Autodesk Inventor part; units mm, degrees
(part 3 of 3)
sketch "Sketch1 outline for Extrusion2" plane through (0, 0, 0) normal (0, 0, 1) x (1, 0, 0)
  arc A0 (21.457911, 5.391973) -> (21.768736, 3.954452) centre (0.000012, -0.000078) cw
  spline S0 degree 3 poles (18.997609, 5.539001) (19.076402, 5.554495) (19.252325, 5.587248) (19.530013, 5.604888) (19.826012, 5.602764) (20.12188, 5.590993) (20.417028, 5.567223) (20.711048, 5.532217) (21.003535, 5.486112) (21.252244, 5.437621) (21.40332, 5.404433) (21.457911, 5.391973) knots 0 0 0 0 0.0970257 0.21631999 0.33564552 0.45497381 0.57430193 0.69363012 0.81295881 0.93228849 1 1 1 1
  spline S1 degree 3 poles (21.768736, 3.954452) (21.724169, 3.920552) (21.600299, 3.827915) (21.39384, 3.681006) (21.146528, 3.518184) (20.893235, 3.364836) (20.634271, 3.221255) (20.369696, 3.088303) (20.101015, 2.964082) (19.840845, 2.865426) (19.667105, 2.822573) (19.588951, 2.804131) knots 0 0 0 0 0.06771151 0.18704119 0.30636988 0.42569807 0.54502619 0.66435448 0.78368001 0.9029743 1 1 1 1
  arc A1 (18.32817, 5.932845) -> (18.997609, 5.539001) centre (18.884737, 6.113009) ccw
  arc A2 (19.588951, 2.804131) -> (19.14202, 2.168903) centre (19.723301, 2.234768) ccw
  arc A3 (18.179447, 6.374019) -> (18.32817, 5.932845) centre (0.000012, -0.000078) cw
  arc A4 (19.14202, 2.168903) -> (19.188845, 1.705696) centre (0.000012, -0.000078) cw
  arc A5 (18.47382, 7.092773) -> (18.179447, 6.374019) centre (18.731497, 6.56758) ccw
  arc A6 (19.188845, 1.705696) -> (19.753861, 1.172762) centre (19.771547, 1.757495) ccw
  spline S2 degree 3 poles (20.342983, 8.6993) (20.307077, 8.656333) (20.206926, 8.538455) (20.038334, 8.349288) (19.833454, 8.135517) (19.620634, 7.92965) (19.400113, 7.732044) (19.171756, 7.543552) (18.937454, 7.362659) (18.70576, 7.208582) (18.545911, 7.128143) (18.47382, 7.092773) knots 0 0 0 0 0.06771151 0.18704119 0.30636988 0.42569807 0.54502619 0.66435448 0.78368001 0.9029743 1 1 1 1
  spline S3 degree 3 poles (19.753861, 1.172762) (19.834125, 1.170334) (20.012926, 1.163119) (20.287577, 1.118526) (20.575682, 1.050589) (20.861513, 0.973276) (21.143972, 0.884426) (21.422831, 0.784871) (21.697725, 0.674838) (21.929408, 0.57222) (22.069312, 0.506247) (22.11976, 0.481952) knots 0 0 0 0 0.0970257 0.21631999 0.33564552 0.45497381 0.57430193 0.69363012 0.81295881 0.93228849 1 1 1 1
  arc A7 (19.720072, 10.031615) -> (20.342983, 8.6993) centre (0.000012, -0.000078) cw
  arc A8 (22.11976, 0.481952) -> (22.102914, -0.988693) centre (0.000012, -0.000078) cw
  spline S4 degree 3 poles (17.288739, 9.627488) (17.362108, 9.660126) (17.526333, 9.731205) (17.793133, 9.810194) (18.082183, 9.873989) (18.373252, 9.92835) (18.66629, 9.970853) (18.960728, 10.00215) (19.256141, 10.022285) (19.509404, 10.030353) (19.664078, 10.031615) (19.720072, 10.031615) knots 0 0 0 0 0.0970257 0.21631999 0.33564552 0.45497381 0.57430193 0.69363012 0.81295881 0.93228849 1 1 1 1
  spline S5 degree 3 poles (22.102914, -0.988693) (22.051921, -1.011826) (21.910543, -1.074577) (21.67657, -1.171861) (21.399228, -1.275568) (21.118162, -1.368709) (20.833741, -1.451065) (20.546215, -1.52181) (20.256629, -1.58313) (19.981028, -1.621419) (19.802109, -1.624537) (19.72181, -1.625125) knots 0 0 0 0 0.06771151 0.18704119 0.30636988 0.42569807 0.54502619 0.66435448 0.78368001 0.9029743 1 1 1 1
  arc A9 (16.548445, 9.862494) -> (17.288739, 9.627488) centre (17.050967, 10.161988) ccw
  arc A10 (19.72181, -1.625125) -> (19.144734, -2.144976) centre (19.726097, -2.210109) ccw
  arc A11 (16.30528, 10.259512) -> (16.548445, 9.862494) centre (0.000012, -0.000078) cw
  arc A12 (19.144734, -2.144976) -> (19.087311, -2.606988) centre (0.000012, -0.000078) cw
  arc A13 (16.432335, 11.025749) -> (16.30528, 10.259512) centre (16.800418, 10.571063) ccw
  arc A14 (19.087311, -2.606988) -> (19.519572, -3.252288) centre (19.66693, -2.686152) ccw
  spline S6 degree 3 poles (17.897148, 13.007925) (17.871704, 12.958046) (17.800294, 12.820837) (17.678023, 12.598898) (17.525848, 12.344896) (17.364174, 12.096835) (17.193153, 11.855112) (17.012465, 11.620532) (16.824289, 11.392037) (16.63269, 11.190266) (16.494749, 11.076275) (16.432335, 11.025749) knots 0 0 0 0 0.06771151 0.18704119 0.30636988 0.42569807 0.54502619 0.66435448 0.78368001 0.9029743 1 1 1 1
  spline S7 degree 3 poles (19.519572, -3.252288) (19.597284, -3.272516) (19.769996, -3.319337) (20.027838, -3.423928) (20.293603, -3.554271) (20.555063, -3.693249) (20.81067, -3.842724) (21.060383, -4.001835) (21.303901, -4.170279) (21.50694, -4.321878) (21.628656, -4.417329) (21.672434, -4.452241) knots 0 0 0 0 0.0970257 0.21631999 0.33564552 0.45497381 0.57430193 0.69363012 0.81295881 0.93228849 1 1 1 1
  arc A15 (16.993387, 14.168226) -> (17.897148, 13.007925) centre (0.000012, -0.000078) cw
  arc A16 (21.672434, -4.452241) -> (21.32876, -5.882265) centre (0.000012, -0.000078) cw
  spline S8 degree 3 poles (14.712939, 13.233209) (14.777206, 13.281355) (14.921497, 13.387194) (15.164031, 13.523572) (15.431639, 13.650087) (15.703314, 13.767854) (15.979547, 13.874499) (16.259638, 13.970529) (16.543164, 14.055895) (16.788282, 14.120117) (16.938797, 14.155766) (16.993387, 14.168226) knots 0 0 0 0 0.0970257 0.21631999 0.33564552 0.45497381 0.57430193 0.69363012 0.81295881 0.93228849 1 1 1 1
  spline S9 degree 3 poles (21.32876, -5.882265) (21.273899, -5.893471) (21.122102, -5.923189) (20.872347, -5.96597) (20.578881, -6.005363) (20.284137, -6.033625) (19.988521, -6.050627) (19.692461, -6.055617) (19.396491, -6.05096) (19.11928, -6.026963) (18.944153, -5.990189) (18.865736, -5.972895) knots 0 0 0 0 0.06771151 0.18704119 0.30636988 0.42569807 0.54502619 0.66435448 0.78368001 0.9029743 1 1 1 1
  arc A17 (13.938913, 13.297591) -> (14.712939, 13.233209) centre (14.362192, 13.701398) ccw
  arc A18 (18.865736, -5.972895) -> (18.187451, -6.3513) centre (18.739744, -6.544166) ccw
  arc A19 (13.6135, 13.630547) -> (13.938913, 13.297591) centre (0.000012, -0.000078) cw
  arc A20 (18.187451, -6.3513) -> (18.02866, -6.788951) centre (0.000012, -0.000078) cw
  arc A21 (13.566865, 14.405845) -> (13.6135, 13.630547) centre (14.026897, 14.044464) ccw
  arc A22 (18.02866, -6.788951) -> (18.306491, -7.514259) centre (18.576131, -6.995107) ccw
  spline S10 degree 3 poles (14.553877, 16.664275) (14.54017, 16.609984) (14.501082, 16.460326) (14.431262, 16.216743) (14.339423, 15.935247) (14.237002, 15.657429) (14.124057, 15.383712) (14.000098, 15.114806) (13.867486, 14.850166) (13.725588, 14.61082) (13.616471, 14.468992) (13.566865, 14.405845) knots 0 0 0 0 0.06771151 0.18704119 0.30636988 0.42569807 0.54502619 0.66435448 0.78368001 0.9029743 1 1 1 1
  spline S11 degree 3 poles (18.306491, -7.514259) (18.377753, -7.551272) (18.535717, -7.635352) (18.763821, -7.794695) (18.993918, -7.980909) (19.217897, -8.174582) (19.433834, -8.377188) (19.641881, -8.587876) (19.841811, -8.806284) (20.006025, -8.999264) (20.10345, -9.119405) (20.138362, -9.163183) knots 0 0 0 0 0.0970257 0.21631999 0.33564552 0.45497381 0.57430193 0.69363012 0.81295881 0.93228849 1 1 1 1
  arc A23 (13.414584, 17.594379) -> (14.553877, 16.664275) centre (0.000012, -0.000078) cw
  arc A24 (20.138362, -9.163183) -> (19.485094, -10.480879) centre (0.000012, -0.000078) cw
  spline S12 degree 3 poles (11.399372, 16.175357) (11.451315, 16.236597) (11.568436, 16.37189) (11.774542, 16.558818) (12.007288, 16.741709) (12.245947, 16.916976) (12.491523, 17.082415) (12.743223, 17.238364) (13.000644, 17.38468) (13.225326, 17.501836) (13.364135, 17.570084) (13.414584, 17.594379) knots 0 0 0 0 0.0970257 0.21631999 0.33564552 0.45497381 0.57430193 0.69363012 0.81295881 0.93228849 1 1 1 1
  spline S13 degree 3 poles (19.485094, -10.480879) (19.429115, -10.479597) (19.27451, -10.474791) (19.021498, -10.460924) (18.726624, -10.434027) (18.432981, -10.395993) (18.140994, -10.346788) (17.851246, -10.285774) (17.563733, -10.215375) (17.298812, -10.130294) (17.136259, -10.055473) (17.063657, -10.021162) knots 0 0 0 0 0.06771151 0.18704119 0.30636988 0.42569807 0.54502619 0.66435448 0.78368001 0.9029743 1 1 1 1
  arc A25 (10.630426, 16.065888) -> (11.399372, 16.175357) centre (10.953237, 16.553759) ccw
  arc A26 (17.063657, -10.021162) -> (16.318174, -10.239147) centre (16.813703, -10.550075) ccw
  arc A27 (10.239082, 16.318084) -> (10.630426, 16.065888) centre (0.000012, -0.000078) cw
  arc A28 (16.318174, -10.239147) -> (16.065978, -10.630492) centre (0.000012, -0.000078) cw
  arc A29 (10.021097, 17.063567) -> (10.239082, 16.318084) centre (10.550009, 16.813614) ccw
  arc A30 (16.065978, -10.630492) -> (16.175447, -11.399438) centre (16.553849, -10.953303) ccw
  spline S14 degree 3 poles (10.480814, 19.485004) (10.479531, 19.429025) (10.474726, 19.274421) (10.460858, 19.021409) (10.433961, 18.726535) (10.395928, 18.432891) (10.346723, 18.140904) (10.285709, 17.851156) (10.215309, 17.563643) (10.130228, 17.298722) (10.055407, 17.136169) (10.021097, 17.063567) knots 0 0 0 0 0.06771151 0.18704119 0.30636988 0.42569807 0.54502619 0.66435448 0.78368001 0.9029743 1 1 1 1
  spline S15 degree 3 poles (16.175447, -11.399438) (16.236686, -11.45138) (16.37198, -11.568502) (16.558907, -11.774608) (16.741799, -12.007354) (16.917066, -12.246012) (17.082505, -12.491589) (17.238454, -12.743289) (17.38477, -13.00071) (17.501926, -13.225392) (17.570173, -13.3642) (17.594468, -13.414649) knots 0 0 0 0 0.0970257 0.21631999 0.33564552 0.45497381 0.57430193 0.69363012 0.81295881 0.93228849 1 1 1 1
  arc A31 (9.163118, 20.138272) -> (10.480814, 19.485004) centre (0.000012, -0.000078) cw
  arc A32 (17.594468, -13.414649) -> (16.664365, -14.553942) centre (0.000012, -0.000078) cw
  spline S16 degree 3 poles (7.514194, 18.306401) (7.551207, 18.377664) (7.635286, 18.535627) (7.794629, 18.763731) (7.980843, 18.993828) (8.174517, 19.217807) (8.377123, 19.433744) (8.58781, 19.641792) (8.806219, 19.841721) (8.999198, 20.005936) (9.11934, 20.10336) (9.163118, 20.138272) knots 0 0 0 0 0.0970257 0.21631999 0.33564552 0.45497381 0.57430193 0.69363012 0.81295881 0.93228849 1 1 1 1
  spline S17 degree 3 poles (16.664365, -14.553942) (16.610074, -14.540235) (16.460416, -14.501148) (16.216833, -14.431328) (15.935337, -14.339489) (15.657519, -14.237067) (15.383802, -14.124123) (15.114896, -14.000164) (14.850256, -13.867551) (14.61091, -13.725654) (14.469082, -13.616536) (14.405934, -13.566931) knots 0 0 0 0 0.06771151 0.18704119 0.30636988 0.42569807 0.54502619 0.66435448 0.78368001 0.9029743 1 1 1 1
  arc A33 (6.788886, 18.02857) -> (7.514194, 18.306401) centre (6.995042, 18.576042) ccw
  arc A34 (14.405934, -13.566931) -> (13.630636, -13.613565) centre (14.044554, -14.026962) ccw
  arc A35 (6.351234, 18.187361) -> (6.788886, 18.02857) centre (0.000012, -0.000078) cw
  arc A36 (13.630636, -13.613565) -> (13.297681, -13.938979) centre (0.000012, -0.000078) cw
  arc A37 (5.972829, 18.865647) -> (6.351234, 18.187361) centre (6.5441, 18.739654) ccw
  arc A38 (13.297681, -13.938979) -> (13.233298, -14.713005) centre (13.701488, -14.362258) ccw
  spline S18 degree 3 poles (5.882199, 21.32867) (5.893406, 21.273809) (5.923123, 21.122012) (5.965904, 20.872258) (6.005297, 20.578791) (6.033559, 20.284047) (6.050561, 19.988431) (6.055552, 19.692372) (6.050895, 19.396401) (6.026898, 19.119191) (5.990123, 18.944064) (5.972829, 18.865647) knots 0 0 0 0 0.06771151 0.18704119 0.30636988 0.42569807 0.54502619 0.66435448 0.78368001 0.9029743 1 1 1 1
  spline S19 degree 3 poles (13.233298, -14.713005) (13.281444, -14.777272) (13.387284, -14.921563) (13.523662, -15.164097) (13.650177, -15.431705) (13.767944, -15.70338) (13.874588, -15.979613) (13.970619, -16.259704) (14.055985, -16.54323) (14.120207, -16.788348) (14.155856, -16.938863) (14.168315, -16.993453) knots 0 0 0 0 0.0970257 0.21631999 0.33564552 0.45497381 0.57430193 0.69363012 0.81295881 0.93228849 1 1 1 1
  arc A39 (4.452175, 21.672344) -> (5.882199, 21.32867) centre (0.000012, -0.000078) cw
  arc A40 (14.168315, -16.993453) -> (13.008015, -17.897214) centre (0.000012, -0.000078) cw
  spline S20 degree 3 poles (3.252223, 19.519482) (3.27245, 19.597194) (3.319271, 19.769907) (3.423862, 20.027749) (3.554205, 20.293513) (3.693183, 20.554973) (3.842659, 20.81058) (4.001769, 21.060294) (4.170213, 21.303811) (4.321813, 21.50685) (4.417263, 21.628566) (4.452175, 21.672344) knots 0 0 0 0 0.0970257 0.21631999 0.33564552 0.45497381 0.57430193 0.69363012 0.81295881 0.93228849 1 1 1 1
  spline S21 degree 3 poles (13.008015, -17.897214) (12.958136, -17.87177) (12.820927, -17.80036) (12.598988, -17.678088) (12.344986, -17.525914) (12.096924, -17.364239) (11.855202, -17.193219) (11.620622, -17.01253) (11.392126, -16.824355) (11.190356, -16.632755) (11.076365, -16.494814) (11.025839, -16.432401) knots 0 0 0 0 0.06771151 0.18704119 0.30636988 0.42569807 0.54502619 0.66435448 0.78368001 0.9029743 1 1 1 1
  arc A41 (2.606923, 19.087221) -> (3.252223, 19.519482) centre (2.686086, 19.66684) ccw
  arc A42 (11.025839, -16.432401) -> (10.259602, -16.305346) centre (10.571152, -16.800484) ccw
  arc A43 (2.14491, 19.144644) -> (2.606923, 19.087221) centre (0.000012, -0.000078) cw
  arc A44 (10.259602, -16.305346) -> (9.862583, -16.548511) centre (0.000012, -0.000078) cw
  arc A45 (1.625059, 19.72172) -> (2.14491, 19.144644) centre (2.210044, 19.726007) ccw
  arc A46 (9.862583, -16.548511) -> (9.627578, -17.288804) centre (10.162077, -17.051033) ccw
  spline S22 degree 3 poles (0.988628, 22.102824) (1.011761, 22.051832) (1.074512, 21.910453) (1.171795, 21.67648) (1.275503, 21.399138) (1.368643, 21.118072) (1.450999, 20.833651) (1.521744, 20.546125) (1.583064, 20.256539) (1.621354, 19.980939) (1.624471, 19.80202) (1.625059, 19.72172) knots 0 0 0 0 0.06771151 0.18704119 0.30636988 0.42569807 0.54502619 0.66435448 0.78368001 0.9029743 1 1 1 1
  spline S23 degree 3 poles (9.627578, -17.288804) (9.660216, -17.362174) (9.731294, -17.526398) (9.810284, -17.793198) (9.874079, -18.082249) (9.928439, -18.373318) (9.970943, -18.666356) (10.002239, -18.960794) (10.022375, -19.256206) (10.030442, -19.50947) (10.031705, -19.664143) (10.031705, -19.720138) knots 0 0 0 0 0.0970257 0.21631999 0.33564552 0.45497381 0.57430193 0.69363012 0.81295881 0.93228849 1 1 1 1
  arc A47 (-0.482018, 22.119671) -> (0.988628, 22.102824) centre (0.000012, -0.000078) cw
  arc A48 (10.031705, -19.720138) -> (8.69939, -20.343048) centre (0.000012, -0.000078) cw
  spline S24 degree 3 poles (-1.172828, 19.753771) (-1.1704, 19.834036) (-1.163185, 20.012837) (-1.118592, 20.287488) (-1.050655, 20.575593) (-0.973342, 20.861423) (-0.884491, 21.143883) (-0.784937, 21.422741) (-0.674904, 21.697635) (-0.572285, 21.929318) (-0.506312, 22.069222) (-0.482018, 22.119671) knots 0 0 0 0 0.0970257 0.21631999 0.33564552 0.45497381 0.57430193 0.69363012 0.81295881 0.93228849 1 1 1 1
  spline S25 degree 3 poles (8.69939, -20.343048) (8.656423, -20.307143) (8.538545, -20.206992) (8.349378, -20.038399) (8.135606, -19.833519) (7.92974, -19.6207) (7.732134, -19.400179) (7.543642, -19.171822) (7.362748, -18.937519) (7.208672, -18.705825) (7.128233, -18.545977) (7.092863, -18.473885) knots 0 0 0 0 0.06771151 0.18704119 0.30636988 0.42569807 0.54502619 0.66435448 0.78368001 0.9029743 1 1 1 1
  arc A49 (-1.705761, 19.188755) -> (-1.172828, 19.753771) centre (-1.75756, 19.771457) ccw
  arc A50 (7.092863, -18.473885) -> (6.374109, -18.179512) centre (6.56767, -18.731562) ccw
  arc A51 (-2.168968, 19.141931) -> (-1.705761, 19.188755) centre (0.000012, -0.000078) cw
  arc A52 (6.374109, -18.179512) -> (5.932935, -18.328236) centre (0.000012, -0.000078) cw
  arc A53 (-2.804197, 19.588861) -> (-2.168968, 19.141931) centre (-2.234833, 19.723211) ccw
  arc A54 (5.932935, -18.328236) -> (5.539091, -18.997675) centre (6.113099, -18.884802) ccw
  spline S26 degree 3 poles (-3.954517, 21.768646) (-3.920617, 21.72408) (-3.82798, 21.600209) (-3.681072, 21.39375) (-3.51825, 21.146438) (-3.364902, 20.893145) (-3.221321, 20.634181) (-3.088369, 20.369606) (-2.964148, 20.100926) (-2.865491, 19.840755) (-2.822639, 19.667016) (-2.804197, 19.588861) knots 0 0 0 0 0.06771151 0.18704119 0.30636988 0.42569807 0.54502619 0.66435448 0.78368001 0.9029743 1 1 1 1
  spline S27 degree 3 poles (5.539091, -18.997675) (5.554585, -19.076467) (5.587338, -19.252391) (5.604978, -19.530079) (5.602854, -19.826078) (5.591082, -20.121946) (5.567313, -20.417094) (5.532306, -20.711114) (5.486201, -21.003601) (5.43771, -21.252309) (5.404523, -21.403386) (5.392063, -21.457976) knots 0 0 0 0 0.0970257 0.21631999 0.33564552 0.45497381 0.57430193 0.69363012 0.81295881 0.93228849 1 1 1 1
  arc A55 (-5.392039, 21.457821) -> (-3.954517, 21.768646) centre (0.000012, -0.000078) cw
  arc A56 (5.392063, -21.457976) -> (3.954541, -21.768801) centre (0.000012, -0.000078) cw
  spline S28 degree 3 poles (-5.539067, 18.99752) (-5.554561, 19.076312) (-5.587313, 19.252235) (-5.604954, 19.529923) (-5.60283, 19.825922) (-5.591058, 20.12179) (-5.567289, 20.416939) (-5.532282, 20.710959) (-5.486177, 21.003445) (-5.437686, 21.252154) (-5.404499, 21.403231) (-5.392039, 21.457821) knots 0 0 0 0 0.0970257 0.21631999 0.33564552 0.45497381 0.57430193 0.69363012 0.81295881 0.93228849 1 1 1 1
  spline S29 degree 3 poles (3.954541, -21.768801) (3.920641, -21.724235) (3.828004, -21.600365) (3.681096, -21.393906) (3.518274, -21.146594) (3.364926, -20.8933) (3.221345, -20.634337) (3.088393, -20.369761) (2.964172, -20.101081) (2.865515, -19.840911) (2.822663, -19.667171) (2.804221, -19.589016) knots 0 0 0 0 0.06771151 0.18704119 0.30636988 0.42569807 0.54502619 0.66435448 0.78368001 0.9029743 1 1 1 1
  arc A57 (-5.932911, 18.328081) -> (-5.539067, 18.99752) centre (-6.113075, 18.884647) ccw
  arc A58 (2.804221, -19.589016) -> (2.168992, -19.142086) centre (2.234857, -19.723366) ccw
  arc A59 (-6.374085, 18.179357) -> (-5.932911, 18.328081) centre (0.000012, -0.000078) cw
  arc A60 (2.168992, -19.142086) -> (1.705785, -19.18891) centre (0.000012, -0.000078) cw
  arc A61 (-7.092838, 18.47373) -> (-6.374085, 18.179357) centre (-6.567646, 18.731407) ccw
  arc A62 (1.705785, -19.18891) -> (1.172852, -19.753927) centre (1.757584, -19.771613) ccw
  spline S30 degree 3 poles (-8.699366, 20.342893) (-8.656399, 20.306988) (-8.538521, 20.206837) (-8.349354, 20.038244) (-8.135582, 19.833364) (-7.929716, 19.620545) (-7.73211, 19.400023) (-7.543618, 19.171666) (-7.362724, 18.937364) (-7.208648, 18.70567) (-7.128209, 18.545822) (-7.092838, 18.47373) knots 0 0 0 0 0.06771151 0.18704119 0.30636988 0.42569807 0.54502619 0.66435448 0.78368001 0.9029743 1 1 1 1
  spline S31 degree 3 poles (1.172852, -19.753927) (1.170424, -19.834191) (1.163209, -20.012992) (1.118616, -20.287643) (1.050679, -20.575748) (0.973366, -20.861578) (0.884515, -21.144038) (0.784961, -21.422896) (0.674928, -21.69779) (0.57231, -21.929473) (0.506337, -22.069377) (0.482042, -22.119826) knots 0 0 0 0 0.0970257 0.21631999 0.33564552 0.45497381 0.57430193 0.69363012 0.81295881 0.93228849 1 1 1 1
  arc A63 (-10.031681, 19.719982) -> (-8.699366, 20.342893) centre (0.000012, -0.000078) cw
  arc A64 (0.482042, -22.119826) -> (-0.988604, -22.102979) centre (0.000012, -0.000078) cw
  spline S32 degree 3 poles (-9.627554, 17.288649) (-9.660192, 17.362018) (-9.73127, 17.526243) (-9.81026, 17.793043) (-9.874055, 18.082094) (-9.928415, 18.373163) (-9.970919, 18.666201) (-10.002215, 18.960638) (-10.022351, 19.256051) (-10.030418, 19.509315) (-10.031681, 19.663988) (-10.031681, 19.719982) knots 0 0 0 0 0.0970257 0.21631999 0.33564552 0.45497381 0.57430193 0.69363012 0.81295881 0.93228849 1 1 1 1
  spline S33 degree 3 poles (-0.988604, -22.102979) (-1.011737, -22.051987) (-1.074487, -21.910609) (-1.171771, -21.676636) (-1.275479, -21.399293) (-1.368619, -21.118227) (-1.450975, -20.833807) (-1.52172, -20.54628) (-1.58304, -20.256694) (-1.62133, -19.981094) (-1.624447, -19.802175) (-1.625035, -19.721876) knots 0 0 0 0 0.06771151 0.18704119 0.30636988 0.42569807 0.54502619 0.66435448 0.78368001 0.9029743 1 1 1 1
  arc A65 (-9.862559, 16.548356) -> (-9.627554, 17.288649) centre (-10.162053, 17.050878) ccw
  arc A66 (-1.625035, -19.721876) -> (-2.144886, -19.144799) centre (-2.21002, -19.726162) ccw
  arc A67 (-10.259578, 16.305191) -> (-9.862559, 16.548356) centre (0.000012, -0.000078) cw
  arc A68 (-2.144886, -19.144799) -> (-2.606899, -19.087376) centre (0.000012, -0.000078) cw
  arc A69 (-11.025815, 16.432245) -> (-10.259578, 16.305191) centre (-10.571128, 16.800328) ccw
  arc A70 (-2.606899, -19.087376) -> (-3.252199, -19.519638) centre (-2.686062, -19.666995) ccw
  spline S34 degree 3 poles (-13.007991, 17.897059) (-12.958112, 17.871614) (-12.820903, 17.800205) (-12.598964, 17.677933) (-12.344962, 17.525758) (-12.0969, 17.364084) (-11.855178, 17.193063) (-11.620598, 17.012375) (-11.392102, 16.8242) (-11.190332, 16.6326) (-11.076341, 16.494659) (-11.025815, 16.432245) knots 0 0 0 0 0.06771151 0.18704119 0.30636988 0.42569807 0.54502619 0.66435448 0.78368001 0.9029743 1 1 1 1
  spline S35 degree 3 poles (-3.252199, -19.519638) (-3.272426, -19.59735) (-3.319247, -19.770062) (-3.423838, -20.027904) (-3.554181, -20.293668) (-3.693159, -20.555129) (-3.842635, -20.810735) (-4.001745, -21.060449) (-4.170189, -21.303966) (-4.321789, -21.507006) (-4.417239, -21.628722) (-4.452151, -21.6725) knots 0 0 0 0 0.0970257 0.21631999 0.33564552 0.45497381 0.57430193 0.69363012 0.81295881 0.93228849 1 1 1 1
  arc A71 (-14.168291, 16.993298) -> (-13.007991, 17.897059) centre (0.000012, -0.000078) cw
  arc A72 (-4.452151, -21.6725) -> (-5.882175, -21.328826) centre (0.000012, -0.000078) cw
  spline S36 degree 3 poles (-13.233274, 14.71285) (-13.28142, 14.777117) (-13.38726, 14.921407) (-13.523638, 15.163941) (-13.650153, 15.431549) (-13.767919, 15.703224) (-13.874564, 15.979457) (-13.970595, 16.259549) (-14.055961, 16.543074) (-14.120183, 16.788193) (-14.155832, 16.938707) (-14.168291, 16.993298) knots 0 0 0 0 0.0970257 0.21631999 0.33564552 0.45497381 0.57430193 0.69363012 0.81295881 0.93228849 1 1 1 1
  spline S37 degree 3 poles (-5.882175, -21.328826) (-5.893381, -21.273964) (-5.923099, -21.122167) (-5.96588, -20.872413) (-6.005273, -20.578947) (-6.033535, -20.284202) (-6.050537, -19.988587) (-6.055528, -19.692527) (-6.050871, -19.396557) (-6.026874, -19.119346) (-5.990099, -18.944219) (-5.972805, -18.865802) knots 0 0 0 0 0.06771151 0.18704119 0.30636988 0.42569807 0.54502619 0.66435448 0.78368001 0.9029743 1 1 1 1
  arc A73 (-13.297657, 13.938823) -> (-13.233274, 14.71285) centre (-13.701464, 14.362102) ccw
  arc A74 (-5.972805, -18.865802) -> (-6.35121, -18.187517) centre (-6.544076, -18.73981) ccw
  arc A75 (-13.630612, 13.61341) -> (-13.297657, 13.938823) centre (0.000012, -0.000078) cw
  arc A76 (-6.35121, -18.187517) -> (-6.788862, -18.028726) centre (0.000012, -0.000078) cw
  arc A77 (-14.40591, 13.566775) -> (-13.630612, 13.61341) centre (-14.04453, 14.026807) ccw
  arc A78 (-6.788862, -18.028726) -> (-7.51417, -18.306557) centre (-6.995018, -18.576197) ccw
  spline S38 degree 3 poles (-16.664341, 14.553787) (-16.61005, 14.54008) (-16.460391, 14.500993) (-16.216809, 14.431172) (-15.935313, 14.339334) (-15.657495, 14.236912) (-15.383777, 14.123968) (-15.114871, 14.000008) (-14.850232, 13.867396) (-14.610886, 13.725498) (-14.469057, 13.616381) (-14.40591, 13.566775) knots 0 0 0 0 0.06771151 0.18704119 0.30636988 0.42569807 0.54502619 0.66435448 0.78368001 0.9029743 1 1 1 1
  spline S39 degree 3 poles (-7.51417, -18.306557) (-7.551183, -18.377819) (-7.635262, -18.535783) (-7.794605, -18.763886) (-7.980819, -18.993983) (-8.174493, -19.217963) (-8.377098, -19.433899) (-8.587786, -19.641947) (-8.806195, -19.841876) (-8.999174, -20.006091) (-9.119316, -20.103515) (-9.163094, -20.138427) knots 0 0 0 0 0.0970257 0.21631999 0.33564552 0.45497381 0.57430193 0.69363012 0.81295881 0.93228849 1 1 1 1
  arc A79 (-17.594444, 13.414494) -> (-16.664341, 14.553787) centre (0.000012, -0.000078) cw
  arc A80 (-9.163094, -20.138427) -> (-10.48079, -19.48516) centre (0.000012, -0.000078) cw
  spline S40 degree 3 poles (-16.175423, 11.399283) (-16.236662, 11.451225) (-16.371956, 11.568346) (-16.558883, 11.774453) (-16.741775, 12.007199) (-16.917042, 12.245857) (-17.082481, 12.491433) (-17.23843, 12.743133) (-17.384746, 13.000555) (-17.501902, 13.225237) (-17.570149, 13.364045) (-17.594444, 13.414494) knots 0 0 0 0 0.0970257 0.21631999 0.33564552 0.45497381 0.57430193 0.69363012 0.81295881 0.93228849 1 1 1 1
  spline S41 degree 3 poles (-10.48079, -19.48516) (-10.479507, -19.42918) (-10.474702, -19.274576) (-10.460834, -19.021564) (-10.433937, -18.72669) (-10.395904, -18.433046) (-10.346699, -18.141059) (-10.285685, -17.851312) (-10.215285, -17.563798) (-10.130204, -17.298878) (-10.055383, -17.136325) (-10.021072, -17.063722) knots 0 0 0 0 0.06771151 0.18704119 0.30636988 0.42569807 0.54502619 0.66435448 0.78368001 0.9029743 1 1 1 1
  arc A81 (-16.065954, 10.630336) -> (-16.175423, 11.399283) centre (-16.553825, 10.953147) ccw
  arc A82 (-10.021072, -17.063722) -> (-10.239058, -16.31824) centre (-10.549985, -16.813769) ccw
  arc A83 (-16.31815, 10.238992) -> (-16.065954, 10.630336) centre (0.000012, -0.000078) cw
  arc A84 (-10.239058, -16.31824) -> (-10.630402, -16.066043) centre (0.000012, -0.000078) cw
  arc A85 (-17.063633, 10.021007) -> (-16.31815, 10.238992) centre (-16.813679, 10.549919) ccw
  arc A86 (-10.630402, -16.066043) -> (-11.399348, -16.175512) centre (-10.953213, -16.553914) ccw
  spline S42 degree 3 poles (-19.48507, 10.480724) (-19.429091, 10.479441) (-19.274486, 10.474636) (-19.021474, 10.460769) (-18.7266, 10.433871) (-18.432957, 10.395838) (-18.140969, 10.346633) (-17.851222, 10.285619) (-17.563709, 10.215219) (-17.298788, 10.130139) (-17.136235, 10.055317) (-17.063633, 10.021007) knots 0 0 0 0 0.06771151 0.18704119 0.30636988 0.42569807 0.54502619 0.66435448 0.78368001 0.9029743 1 1 1 1
  spline S43 degree 3 poles (-11.399348, -16.175512) (-11.451291, -16.236752) (-11.568412, -16.372046) (-11.774518, -16.558973) (-12.007264, -16.741865) (-12.245922, -16.917132) (-12.491499, -17.08257) (-12.743199, -17.238519) (-13.00062, -17.384836) (-13.225302, -17.501991) (-13.364111, -17.570239) (-13.41456, -17.594534) knots 0 0 0 0 0.0970257 0.21631999 0.33564552 0.45497381 0.57430193 0.69363012 0.81295881 0.93228849 1 1 1 1
  arc A87 (-20.138338, 9.163028) -> (-19.48507, 10.480724) centre (0.000012, -0.000078) cw
  arc A88 (-13.41456, -17.594534) -> (-14.553853, -16.66443) centre (0.000012, -0.000078) cw
  spline S44 degree 3 poles (-18.306467, 7.514104) (-18.377729, 7.551117) (-18.535693, 7.635196) (-18.763797, 7.79454) (-18.993894, 7.980753) (-19.217873, 8.174427) (-19.43381, 8.377033) (-19.641857, 8.58772) (-19.841787, 8.806129) (-20.006001, 8.999108) (-20.103426, 9.11925) (-20.138338, 9.163028) knots 0 0 0 0 0.0970257 0.21631999 0.33564552 0.45497381 0.57430193 0.69363012 0.81295881 0.93228849 1 1 1 1
  spline S45 degree 3 poles (-14.553853, -16.66443) (-14.540146, -16.61014) (-14.501058, -16.460481) (-14.431238, -16.216898) (-14.339399, -15.935403) (-14.236978, -15.657585) (-14.124033, -15.383867) (-14.000074, -15.114961) (-13.867462, -14.850322) (-13.725564, -14.610975) (-13.616447, -14.469147) (-13.566841, -14.406) knots 0 0 0 0 0.06771151 0.18704119 0.30636988 0.42569807 0.54502619 0.66435448 0.78368001 0.9029743 1 1 1 1
  arc A89 (-18.028636, 6.788796) -> (-18.306467, 7.514104) centre (-18.576107, 6.994952) ccw
  arc A90 (-13.566841, -14.406) -> (-13.613476, -13.630702) centre (-14.026873, -14.044619) ccw
  arc A91 (-18.187427, 6.351145) -> (-18.028636, 6.788796) centre (0.000012, -0.000078) cw
  arc A92 (-13.613476, -13.630702) -> (-13.938889, -13.297747) centre (0.000012, -0.000078) cw
  arc A93 (-18.865712, 5.972739) -> (-18.187427, 6.351145) centre (-18.73972, 6.544011) ccw
  arc A94 (-13.938889, -13.297747) -> (-14.712915, -13.233364) centre (-14.362168, -13.701553) ccw
  spline S46 degree 3 poles (-21.328736, 5.88211) (-21.273875, 5.893316) (-21.122078, 5.923034) (-20.872323, 5.965815) (-20.578857, 6.005207) (-20.284113, 6.033469) (-19.988497, 6.050471) (-19.692437, 6.055462) (-19.396467, 6.050805) (-19.119256, 6.026808) (-18.944129, 5.990034) (-18.865712, 5.972739) knots 0 0 0 0 0.06771151 0.18704119 0.30636988 0.42569807 0.54502619 0.66435448 0.78368001 0.9029743 1 1 1 1
  spline S47 degree 3 poles (-14.712915, -13.233364) (-14.777182, -13.28151) (-14.921473, -13.38735) (-15.164007, -13.523727) (-15.431615, -13.650243) (-15.70329, -13.768009) (-15.979523, -13.874654) (-16.259614, -13.970684) (-16.54314, -14.056051) (-16.788258, -14.120272) (-16.938773, -14.155921) (-16.993363, -14.168381) knots 0 0 0 0 0.0970257 0.21631999 0.33564552 0.45497381 0.57430193 0.69363012 0.81295881 0.93228849 1 1 1 1
  arc A95 (-21.67241, 4.452085) -> (-21.328736, 5.88211) centre (0.000012, -0.000078) cw
  arc A96 (-16.993363, -14.168381) -> (-17.897124, -13.008081) centre (0.000012, -0.000078) cw
  spline S48 degree 3 poles (-19.519548, 3.252133) (-19.59726, 3.272361) (-19.769972, 3.319182) (-20.027814, 3.423772) (-20.293579, 3.554116) (-20.555039, 3.693093) (-20.810645, 3.842569) (-21.060359, 4.001679) (-21.303877, 4.170124) (-21.506916, 4.321723) (-21.628632, 4.417174) (-21.67241, 4.452085) knots 0 0 0 0 0.0970257 0.21631999 0.33564552 0.45497381 0.57430193 0.69363012 0.81295881 0.93228849 1 1 1 1
  spline S49 degree 3 poles (-17.897124, -13.008081) (-17.87168, -12.958201) (-17.80027, -12.820993) (-17.677999, -12.599054) (-17.525824, -12.345052) (-17.36415, -12.09699) (-17.193129, -11.855268) (-17.012441, -11.620687) (-16.824265, -11.392192) (-16.632666, -11.190422) (-16.494725, -11.07643) (-16.432311, -11.025905) knots 0 0 0 0 0.06771151 0.18704119 0.30636988 0.42569807 0.54502619 0.66435448 0.78368001 0.9029743 1 1 1 1
  arc A97 (-19.087287, 2.606833) -> (-19.519548, 3.252133) centre (-19.666906, 2.685996) ccw
  arc A98 (-16.432311, -11.025905) -> (-16.305256, -10.259668) centre (-16.800394, -10.571218) ccw
  arc A99 (-19.14471, 2.14482) -> (-19.087287, 2.606833) centre (0.000012, -0.000078) cw
  arc A100 (-16.305256, -10.259668) -> (-16.548421, -9.862649) centre (0.000012, -0.000078) cw
  arc A101 (-19.721786, 1.62497) -> (-19.14471, 2.14482) centre (-19.726073, 2.209954) ccw
  arc A102 (-16.548421, -9.862649) -> (-17.288715, -9.627643) centre (-17.050943, -10.162143) ccw
  spline S50 degree 3 poles (-22.10289, 0.988538) (-22.051897, 1.011671) (-21.910519, 1.074422) (-21.676546, 1.171706) (-21.399204, 1.275413) (-21.118138, 1.368553) (-20.833717, 1.45091) (-20.546191, 1.521655) (-20.256605, 1.582974) (-19.981004, 1.621264) (-19.802085, 1.624381) (-19.721786, 1.62497) knots 0 0 0 0 0.06771151 0.18704119 0.30636988 0.42569807 0.54502619 0.66435448 0.78368001 0.9029743 1 1 1 1
  spline S51 degree 3 poles (-17.288715, -9.627643) (-17.362084, -9.660282) (-17.526309, -9.73136) (-17.793109, -9.81035) (-18.082159, -9.874144) (-18.373228, -9.928505) (-18.666266, -9.971008) (-18.960704, -10.002305) (-19.256117, -10.02244) (-19.50938, -10.030508) (-19.664054, -10.03177) (-19.720048, -10.03177) knots 0 0 0 0 0.0970257 0.21631999 0.33564552 0.45497381 0.57430193 0.69363012 0.81295881 0.93228849 1 1 1 1
  arc A103 (-22.119736, -0.482107) -> (-22.10289, 0.988538) centre (0.000012, -0.000078) cw
  arc A104 (-19.720048, -10.03177) -> (-20.342959, -8.699455) centre (0.000012, -0.000078) cw
  spline S52 degree 3 poles (-19.753837, -1.172917) (-19.834101, -1.17049) (-20.012902, -1.163275) (-20.287553, -1.118681) (-20.575658, -1.050744) (-20.861489, -0.973431) (-21.143948, -0.884581) (-21.422807, -0.785027) (-21.697701, -0.674993) (-21.929384, -0.572375) (-22.069287, -0.506402) (-22.119736, -0.482107) knots 0 0 0 0 0.0970257 0.21631999 0.33564552 0.45497381 0.57430193 0.69363012 0.81295881 0.93228849 1 1 1 1
  spline S53 degree 3 poles (-20.342959, -8.699455) (-20.307053, -8.656489) (-20.206902, -8.53861) (-20.03831, -8.349443) (-19.83343, -8.135672) (-19.62061, -7.929806) (-19.400089, -7.7322) (-19.171732, -7.543707) (-18.93743, -7.362814) (-18.705736, -7.208737) (-18.545887, -7.128299) (-18.473796, -7.092928) knots 0 0 0 0 0.06771151 0.18704119 0.30636988 0.42569807 0.54502619 0.66435448 0.78368001 0.9029743 1 1 1 1
  arc A105 (-19.188821, -1.705851) -> (-19.753837, -1.172917) centre (-19.771523, -1.75765) ccw
  arc A106 (-18.473796, -7.092928) -> (-18.179423, -6.374175) centre (-18.731473, -6.567735) ccw
  arc A107 (-19.141996, -2.169058) -> (-19.188821, -1.705851) centre (0.000012, -0.000078) cw
  arc A108 (-18.179423, -6.374175) -> (-18.328146, -5.933001) centre (0.000012, -0.000078) cw
  arc A109 (-19.588926, -2.804287) -> (-19.141996, -2.169058) centre (-19.723277, -2.234923) ccw
  arc A110 (-18.328146, -5.933001) -> (-18.997585, -5.539157) centre (-18.884713, -6.113164) ccw
  spline S54 degree 3 poles (-21.768711, -3.954607) (-21.724145, -3.920707) (-21.600275, -3.82807) (-21.393816, -3.681161) (-21.146504, -3.51834) (-20.893211, -3.364992) (-20.634247, -3.22141) (-20.369672, -3.088459) (-20.100991, -2.964238) (-19.840821, -2.865581) (-19.667081, -2.822729) (-19.588926, -2.804287) knots 0 0 0 0 0.06771151 0.18704119 0.30636988 0.42569807 0.54502619 0.66435448 0.78368001 0.9029743 1 1 1 1
  spline S55 degree 3 poles (-18.997585, -5.539157) (-19.076378, -5.55465) (-19.252301, -5.587403) (-19.529989, -5.605044) (-19.825988, -5.602919) (-20.121856, -5.591148) (-20.417004, -5.567379) (-20.711024, -5.532372) (-21.003511, -5.486267) (-21.25222, -5.437776) (-21.403296, -5.404589) (-21.457887, -5.392129) knots 0 0 0 0 0.0970257 0.21631999 0.33564552 0.45497381 0.57430193 0.69363012 0.81295881 0.93228849 1 1 1 1
  arc A111 (-21.457887, -5.392129) -> (-21.768711, -3.954607) centre (0.000012, -0.000078) cw
  circle A112 centre (-6.472069, -4.702415) radius 2.5
  circle A113 centre (0.000012, -0.000078) radius 3.5
  circle A114 centre (2.472218, -7.608494) radius 2.5
  circle A115 centre (-6.47216, 4.702134) radius 2.5
  circle A116 centre (8, 0) radius 2.5
  circle A117 centre (2.47207, 7.608387) radius 2.5
extrude "Extrusion2" add sketch "Sketch1 outline for Extrusion2" along normal blind 10
body "Solid2"
